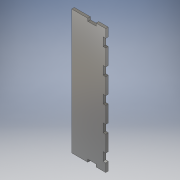
# Autodesk Inventor part: 1-8inch_Bottom2_1-Part
Saved by Autodesk Inventor 2018 (Build 220112000, 112)
## iProperties
Created: 2018-02-01
Part Number: 1-8inch_Bottom2_1-Part
Material: Generic
Document SubType Name: Modeling
Designer: Angie
Density: 1 g/cm^3
Appearance: Default
Author: Angie
Autodesk Inventor part; units mm, degrees
ref_plane "YZ Plane" through (0, 0, 0) normal (1, 0, 0) x (0, 1, 0)
ref_plane "XZ Plane" through (0, 0, 0) normal (0, 1, 0) x (-1, 0, 0)
ref_plane "XY Plane" through (0, 0, 0) normal (0, 0, 1) x (1, 0, 0)
sketch "Sketch1" plane through (0, 0, 0) normal (0, 0, 1) x (1, 0, 0)
  line L0 (-11.5, -148.5) -> (-11.5, -147.1375)
  line L1 (-21.5, -147.1375) -> (-21.5, -148.5)
  line L2 (-41, -148.5) -> (-41, 0.5)
  line L3 (-41, 0.5) -> (-21.5, 0.5)
  line L4 (-21.5, 0.5) -> (-21.5, -2.5)
  line L5 (-11.5, -2.5) -> (-11.5, 0.5)
  line L6 (-11.5, 0.5) -> (0, 0.5)
  line L7 (-11.5, -148.5) -> (-11.5, -147.1375)
  line L8 (-21.5, -147.1375) -> (-21.5, -148.5)
  line L9 (-41, -148.5) -> (-41, 0.5)
  line L10 (-41, 0.5) -> (-21.5, 0.5)
  line L11 (-21.5, 0.5) -> (-21.5, -2.5)
  line L12 (-11.5, -2.5) -> (-11.5, 0.5)
  line L13 (-11.5, 0.5) -> (0, 0.5)
  line L14 (-41, -150.3125) -> (-41, 0.5)
  line L15 (-11.5, -150.3125) -> (-11.5, -147.1375)
  line L16 (-11.5, -147.1375) -> (-21.5, -147.1375)
  line L17 (-21.5, -147.1375) -> (-21.5, -150.3125)
  line L18 (0, -150.3125) -> (-11.5, -150.3125)
  line L19 (-21.5, -150.3125) -> (-41, -150.3125)
  line L20 (-11.5, 0.5) -> (-11.5, -2.675)
  line L21 (-11.5, -2.675) -> (-21.5, -2.675)
  line L22 (-21.5, -2.675) -> (-21.5, 0.5)
  line L23 (0, 0.5) -> (-3.175, 0.5)
  line L24 (-3.175, -150.3125) -> (0, -150.3125)
  line L25 (-3.175, 0.5) -> (0, 0.5)
  line L26 (0, -9.66) -> (-2.9986, -9.66)
  line L27 (-2.9986, -9.66) -> (0, -9.66)
  line L28 (0, -19.82) -> (-2.9986, -19.82)
  line L29 (-2.9986, -19.82) -> (0, -19.82)
  line L30 (0, -39.7431) -> (-2.9986, -39.7431)
  line L31 (-2.9986, -39.7431) -> (0, -39.7431)
  line L32 (0, -49.9031) -> (-2.9986, -49.9031)
  line L33 (-2.9986, -49.9031) -> (0, -49.9031)
  line L34 (0, -69.8263) -> (-2.9986, -69.8263)
  line L35 (-2.9986, -69.8263) -> (0, -69.8263)
  line L36 (0, -79.9863) -> (-2.9986, -79.9863)
  line L37 (-2.9986, -79.9863) -> (0, -79.9863)
  line L38 (0, -99.9094) -> (-2.9986, -99.9094)
  line L39 (-2.9986, -99.9094) -> (0, -99.9094)
  line L40 (0, -110.0694) -> (-2.9986, -110.0694)
  line L41 (-2.9986, -110.0694) -> (0, -110.0694)
  line L42 (0, -129.9925) -> (-2.9986, -129.9925)
  line L43 (-2.9986, -129.9925) -> (0, -129.9925)
  line L44 (0, -140.1525) -> (-2.9986, -140.1525)
  line L45 (-2.9986, -140.1525) -> (0, -140.1525)
  line L46 (0, -150.3125) -> (-3.175, -150.3125)
  line L47 (-41, 0.5) -> (-21.5, 0.5)
  line L48 (-11.5, 0.5) -> (0, 0.5)
  line L49 (-2.9986, -9.66) -> (-2.9986, -19.82)
  line L50 (-2.9986, -39.7431) -> (-2.9986, -49.9031)
  line L51 (0, -49.9031) -> (0.1778, -49.9031)
  line L52 (0.1778, -49.9031) -> (0.1778, -69.8263)
  line L53 (0.1778, -69.8263) -> (0, -69.8263)
  line L54 (-2.9986, -69.8263) -> (-2.9986, -79.9863)
  line L55 (0, -79.9863) -> (0.1778, -79.9863)
  line L56 (0.1778, -79.9863) -> (0.1778, -99.9094)
  line L57 (0.1778, -99.9094) -> (0, -99.9094)
  line L58 (-2.9986, -99.9094) -> (-2.9986, -110.0694)
  line L59 (-2.9986, -129.9925) -> (-2.9986, -140.1525)
  line L60 (0.1778, -150.3125) -> (0, -150.3125)
  line L61 (0, -140.1525) -> (0.1778, -140.1525)
  line L62 (0, -129.9925) -> (0.1778, -129.9925)
  line L63 (0, -110.0694) -> (0.1778, -110.0694)
  line L64 (0.1778, -110.0694) -> (0.1778, -129.9925)
  line L65 (0.1778, -140.1525) -> (0.1778, -150.3125)
  line L66 (0, -39.7431) -> (0.1778, -39.7431)
  line L67 (0.1778, -39.7431) -> (0.1778, -19.82)
  line L68 (0.1778, -19.82) -> (0, -19.82)
  line L69 (0, -9.66) -> (0.1778, -9.66)
  line L70 (0.1778, -9.66) -> (0.1778, 0.5)
  line L71 (0.1778, 0.5) -> (0, 0.5)
  point P0 (0, 0)
  dimension "d2" = 3.175
  dimension "d4" = 10.16
  dimension "d5" = 10.16
  dimension "d6" = 19.9231
  dimension "d7" = 10.16
  dimension "d8" = 19.9231
  dimension "d9" = 10.16
  dimension "d10" = 19.9231
  dimension "d13" = 10.16
  constraints: 144 end point, 21 parallel, 17 horizontal, 12 perpendicular, 11 point on line
  measures "d2" distance of L5.end L20.end
  measures "d4" distance of L6.end L26.start
  measures "d5" distance of L28.start L26.start
  measures "d6" distance of L28.start L30.start
  measures "d7" distance of L32.start L30.start
  measures "d8" distance of L34.start L32.start
  measures "d9" distance of L34.start L36.start
  measures "d10" distance of L38.start L36.start
  measures "d13" distance of L42.start L44.start
extrude "Extrusion2" add sketch "Sketch1" along normal blind 3.175
body "Solid2"
